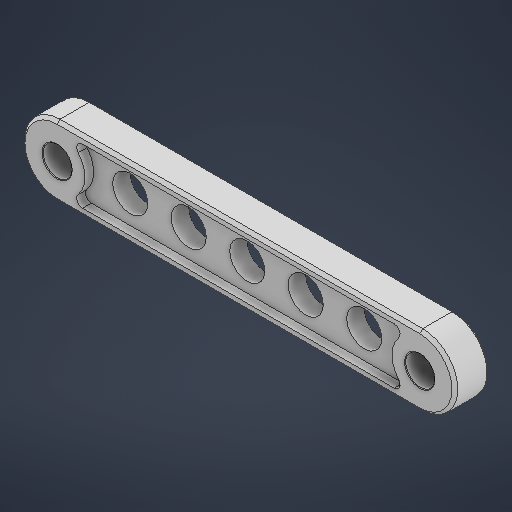
# Autodesk Inventor part: Crankrod
Saved by Autodesk Inventor 2025.4 (Build 294407000, 407)
## iProperties
Created: 2026-05-29
Part Number: Crankrod
Material: Generic
Document SubType Name: Modeling
Designer: VuQuan
Density: 1 g/cm^3
Appearance: Default
Author: VuQuan
Autodesk Inventor part; units mm, degrees
ref_plane "YZ Plane" through (0, 0, 0) normal (1, 0, 0) x (0, 1, 0)
ref_plane "XZ Plane" through (0, 0, 0) normal (0, 1, 0) x (-1, 0, 0)
ref_plane "XY Plane" through (0, 0, 0) normal (0, 0, 1) x (1, 0, 0)
sketch "Sketch1" plane through (0, 0, 0) normal (0, 0, 1) x (1, 0, 0)
  line L0 (0, 0) -> (62, 0) construction
  line L1 (0, -6) -> (62, -6)
  line L2 (62, 6) -> (0, 6)
  arc A0 (0, 6) -> (0, -6) centre (0, 0) ccw
  arc A1 (62, -6) -> (62, 6) centre (62, 0) ccw
  circle A2 centre (0, 0) radius 2.5
  circle A3 centre (62, 0) radius 2.5
  circle A4 centre (11, 0) radius 3
  circle A5 centre (21, 0) radius 3
  circle A6 centre (31, 0) radius 3
  circle A7 centre (41, 0) radius 3
  circle A8 centre (51, 0) radius 3
  point P0 (31, 0)
  dimension "d0" = 6
  dimension "d1" = 5
  dimension "d2" = 62
  dimension "d3" = 6
  dimension "d4" = 11
  dimension "d7" = 10
  constraints: 9 centre point, 8 end point, 4 point on circle, 4 tangent, 2 coincident, 2 horizontal, 1 equal radius, 1 midpoint, 1 parallel, 1 point on line, 8 other
  measures "d0" radius of A0
  measures "d1" diameter of A2
  measures "d2" distance of L0.end L0.start
  measures "d3" diameter of A4
  measures "d4" distance of L0.start A4.centre
  measures "d7" distance of A4.centre A5.centre
extrude "Extrusion1" add sketch "Sketch1" along normal mid plane 6
sketch "Sketch2" plane through (0, 0, 3) normal (0, 0, 1) x (1, 0, 0)
  arc A0 (0, 6) -> (0, -6) centre (0, 0) ccw projected
  circle A1 centre (11, 0) radius 3 projected
  circle A2 centre (21, 0) radius 3 projected
  circle A3 centre (31, 0) radius 3 projected
  circle A4 centre (41, 0) radius 3 projected
  circle A5 centre (51, 0) radius 3 projected
  line L0 (4.3589, 4.75) -> (57.6411, 4.75)
  line L1 (57.6411, -4.75) -> (4.3589, -4.75)
  arc A6 (3.6008, -3.0978) -> (3.6008, 3.0978) centre (0, 0) ccw
  arc A7 (4.3589, 4.75) -> (3.6008, 3.0978) centre (4.3589, 3.75) ccw
  arc A8 (3.6008, -3.0978) -> (4.3589, -4.75) centre (4.3589, -3.75) ccw
  line L2 (31, 3) -> (31, -3) construction
  arc A9 (58.3992, 3.0978) -> (58.3992, -3.0978) centre (62, 0) ccw
  arc A10 (57.6411, -4.75) -> (58.3992, -3.0978) centre (57.6411, -3.75) ccw
  arc A11 (58.3992, 3.0978) -> (57.6411, 4.75) centre (57.6411, 3.75) ccw
  point P0 (0, 4.75)
  point P1 (0, -4.75)
  dimension "d14" = 1
  dimension "d15" = 4.75
  constraints: 16 point on circle, 7 symmetric about line, 6 centre point, 6 end point, 6 tangent, 2 coincident, 2 horizontal, 2 point on line, 1 equal radius, 1 midpoint, 1 vertical, 3 other
  measures "d14" radius of A7
  measures "d15" radius of A6
extrude "Extrusion2" cut sketch "Sketch2" against normal blind 1.5
mirror "Mirror1" about plane through (0, 0, 0) normal (0, 0, 1) of "Extrusion2"
chamfer "Chamfer1" distance 0.5 angle 45 8 edges at (31, 6, 3) (-6, 0, 3) (31, -6, 3) (68, 0, 3) (31, 6, -3) (68, 0, -3) (31, -6, -3) (-6, 0, -3)
chamfer "Chamfer2" distance 0.1 angle 45 4 edges at (-2.5, 0, 3) (59.5, 0, 3) (59.5, 0, -3) (-2.5, 0, -3)
ref_plane "Work Plane1" through (0, 0, 0) normal (0, 0, 1) x (1, 0, 0)
body "Solid1"
